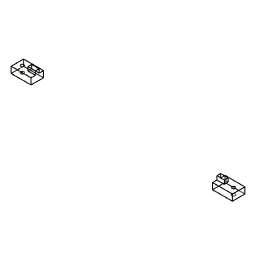
_Drawslide Aligning Spacer (Autodesk Fusion 360 design; units mm, degrees)
Autodesk Fusion 360 part; units mm, degrees
ref_plane "WorkPlane1" through (0, 0, 160) normal (0, 0, 1) x (1, 0, 0)
sketch "Sketch1" plane through (0, 0, 160) normal (0, 0, 1) x (1, 0, 0)
  circle A0 centre (314.6846, 40) radius 2.5
  line L0 (322.6846, 50) -> (302.6846, 50)
  line L1 (302.6846, 50) -> (302.6846, 30)
  line L2 (302.6846, 30) -> (322.6846, 30)
  line L3 (322.6846, 30) -> (322.6846, 50)
  circle A1 centre (-24.6846, 40) radius 2.5
  line L4 (-32.6846, 30) -> (-12.6846, 30)
  line L5 (-12.6846, 30) -> (-12.6846, 50)
  line L6 (-12.6846, 50) -> (-32.6846, 50)
  line L7 (-32.6846, 50) -> (-32.6846, 30)
  line L8 (-32.6846, 50) -> (322.6846, 50)
  line L9 (322.6846, 50) -> (322.6846, 30)
  line L10 (322.6846, 30) -> (-32.6846, 30)
  line L11 (-32.6846, 30) -> (-32.6846, 50)
  line L12 (145, 30) -> (145, 50)
  line L13 (-0.6846, 50) -> (-0.6846, 30)
  line L14 (290.6846, 50) -> (290.6846, 30)
  dimension "d281" = 12
  constraint horizontal L8
  constraint vertical L9
  constraint horizontal L10
  constraint vertical L11
  constraint coincident L2.end L3.start
  constraint coincident L6.end L7.start
  constraint midpoint L10 L12.start
  constraint midpoint L8 L12.end
  constraint coincident L8 L13.start
  constraint coincident L10 L13.end
  constraint perpendicular L10 L13
  constraint symmetric L12 L13.start L14.start
  constraint symmetric L12 L13.end L14.end
  measures "d281" distance of L5 L13
extrude "Extrude1" add sketch "Sketch1" against normal blind 10 contours L0 L1 L2 L3 L8 L9 L10 | L1 L8 L10 L14 | L5 L8 L10 L13 | L4 L5 L6 L7 L8 L10 L11 makes body 1 at (-7.8513, 40, 160) makes body 2 at (297.8513, 40, 160)
sketch "Sketch2" plane through (0, 0, 160) normal (0, 0, 1) x (-1, 0, 0)
  circle A0 centre (24.6846, -40) radius 2.5
  line L0 (0.6846, -50) -> (32.6846, -50)
  line L1 (32.6846, -50) -> (32.6846, -30)
  line L2 (32.6846, -30) -> (0.6846, -30)
  circle A1 centre (-314.6846, -40) radius 2.5
  line L3 (-290.6846, -30) -> (-322.6846, -30)
  line L4 (-322.6846, -30) -> (-322.6846, -50)
  line L5 (-322.6846, -50) -> (-290.6846, -50)
  line L6 (0.6846, -43) -> (12.6846, -43)
  line L7 (12.6846, -43) -> (12.6846, -37)
  line L8 (12.6846, -37) -> (0.6846, -37)
  line L9 (0.6846, -37) -> (0.6846, -43)
  line L10 (12.6846, -40) -> (32.6846, -40)
  line L11 (-145, -30) -> (-145, -50)
  line L12 (-290.6846, -43) -> (-302.6846, -43)
  line L13 (-302.6846, -43) -> (-302.6846, -37)
  line L14 (-290.6846, -37) -> (-290.6846, -43)
  line L15 (-302.6846, -37) -> (-290.6846, -37)
  line L16 (0.6846, -30) -> (0.6846, -50)
  line L17 (-290.6846, -50) -> (-290.6846, -30)
  dimension "d277" = 6
  dimension "d278" = 12
  constraint horizontal L6
  constraint vertical L7
  constraint horizontal L8
  constraint vertical L9
  constraint midpoint L7 L10.start
  constraint perpendicular L7 L10
  constraint midpoint L1 L10.end
  constraint symmetric L6.start L11 L12.start
  constraint symmetric L6.end L11 L12.end
  constraint symmetric L7.end L11 L13.end
  constraint symmetric L8.end L11 L14.start
  constraint coincident L6.start L16
  measures "d277" distance of L6.end L7.end
  measures "d278" distance of L6.start L6.end
extrude "Extrude2" add sketch "Sketch2" along normal blind 6 contours L6 L7 L8 L9 L16 | L12 L13 L14 L15 L17 bodies 1 2
equation "d274 = drawerHeight + 2 * thicknessMDF"
equation "d275 = -thicknessMDF"
equation "drawerHeight = 160 mm - 2 * thicknessMDF"
equation "thicknessMDF = 10 mm"
